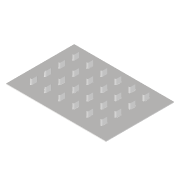
# Autodesk Inventor part: 00_Omniscope_PCB_USBC
Saved by Autodesk Inventor 2022 (Build 260153000, 153)
## iProperties
Created: 2023-05-17
Part Number: 00_Omniscope_PCB_USBC
Material: Generisch
Document SubType Name: Modeling
Designer: diederichbenedict
Density: 1 g/cm^3
Appearance: Vorgabe
Author: diederichbenedict
Autodesk Inventor part; units mm, degrees
(part 1 of 5)
ref_plane "YZ Plane" through (0, 0, 0) normal (1, 0, 0) x (0, 1, 0)
ref_plane "XZ Plane" through (0, 0, 0) normal (0, 1, 0) x (-1, 0, 0)
ref_plane "XY Plane" through (0, 0, 0) normal (0, 0, 1) x (1, 0, 0)
sketch "Skizze5" plane through (0, 0, 0) normal (0, 1, 0) x (-1, 0, 0)
  line L0 (78.8326, 37.2618) -> (79.6226, 37.2618)
  line L1 (79.6226, 37.2618) -> (79.6226, 36.8618)
  line L2 (79.6226, 36.8618) -> (78.8326, 36.8618)
  line L3 (78.8326, 36.8618) -> (78.8326, 37.2618)
  line L4 (76.2926, 37.2618) -> (77.0826, 37.2618)
  line L5 (77.0826, 37.2618) -> (77.0826, 36.8618)
  line L6 (77.0826, 36.8618) -> (76.2926, 36.8618)
  line L7 (76.2926, 36.8618) -> (76.2926, 37.2618)
  line L8 (78.8326, 36.4618) -> (79.6226, 36.4618)
  line L9 (79.6226, 36.4618) -> (79.6226, 36.0618)
  line L10 (79.6226, 36.0618) -> (78.8326, 36.0618)
  line L11 (78.8326, 36.0618) -> (78.8326, 36.4618)
  line L12 (76.2926, 36.4618) -> (77.0826, 36.4618)
  line L13 (77.0826, 36.4618) -> (77.0826, 36.0618)
  line L14 (77.0826, 36.0618) -> (76.2926, 36.0618)
  line L15 (76.2926, 36.0618) -> (76.2926, 36.4618)
  line L16 (78.8326, 35.6618) -> (79.6226, 35.6618)
  line L17 (79.6226, 35.6618) -> (79.6226, 35.2618)
  line L18 (79.6226, 35.2618) -> (78.8326, 35.2618)
  line L19 (78.8326, 35.2618) -> (78.8326, 35.6618)
  line L20 (76.2926, 35.6618) -> (77.0826, 35.6618)
  line L21 (77.0826, 35.6618) -> (77.0826, 35.2618)
  line L22 (77.0826, 35.2618) -> (76.2926, 35.2618)
  line L23 (76.2926, 35.2618) -> (76.2926, 35.6618)
  line L24 (78.8326, 34.8618) -> (79.6226, 34.8618)
  line L25 (79.6226, 34.8618) -> (79.6226, 34.4618)
  line L26 (79.6226, 34.4618) -> (78.8326, 34.4618)
  line L27 (78.8326, 34.4618) -> (78.8326, 34.8618)
  line L28 (76.2926, 34.8618) -> (77.0826, 34.8618)
  line L29 (77.0826, 34.8618) -> (77.0826, 34.4618)
  line L30 (77.0826, 34.4618) -> (76.2926, 34.4618)
  line L31 (76.2926, 34.4618) -> (76.2926, 34.8618)
  line L32 (78.8326, 34.0618) -> (79.6226, 34.0618)
  line L33 (79.6226, 34.0618) -> (79.6226, 33.6618)
  line L34 (79.6226, 33.6618) -> (78.8326, 33.6618)
  line L35 (78.8326, 33.6618) -> (78.8326, 34.0618)
  line L36 (76.2926, 34.0618) -> (77.0826, 34.0618)
  line L37 (77.0826, 34.0618) -> (77.0826, 33.6618)
  line L38 (77.0826, 33.6618) -> (76.2926, 33.6618)
  line L39 (76.2926, 33.6618) -> (76.2926, 34.0618)
  line L40 (78.8326, 33.2618) -> (79.6226, 33.2618)
  line L41 (79.6226, 33.2618) -> (79.6226, 32.8618)
  line L42 (79.6226, 32.8618) -> (78.8326, 32.8618)
  line L43 (78.8326, 32.8618) -> (78.8326, 33.2618)
  line L44 (76.2926, 33.2618) -> (77.0826, 33.2618)
  line L45 (77.0826, 33.2618) -> (77.0826, 32.8618)
  line L46 (77.0826, 32.8618) -> (76.2926, 32.8618)
  line L47 (76.2926, 32.8618) -> (76.2926, 33.2618)
  line L48 (78.8326, 32.4618) -> (79.6226, 32.4618)
  line L49 (79.6226, 32.4618) -> (79.6226, 32.0618)
  line L50 (79.6226, 32.0618) -> (78.8326, 32.0618)
  line L51 (78.8326, 32.0618) -> (78.8326, 32.4618)
  line L52 (76.2926, 32.4618) -> (77.0826, 32.4618)
  line L53 (77.0826, 32.4618) -> (77.0826, 32.0618)
  line L54 (77.0826, 32.0618) -> (76.2926, 32.0618)
  line L55 (76.2926, 32.0618) -> (76.2926, 32.4618)
  line L56 (78.8326, 31.6618) -> (79.6226, 31.6618)
  line L57 (79.6226, 31.6618) -> (79.6226, 31.2618)
  line L58 (79.6226, 31.2618) -> (78.8326, 31.2618)
  line L59 (78.8326, 31.2618) -> (78.8326, 31.6618)
  line L60 (76.2926, 31.6618) -> (77.0826, 31.6618)
  line L61 (77.0826, 31.6618) -> (77.0826, 31.2618)
  line L62 (77.0826, 31.2618) -> (76.2926, 31.2618)
  line L63 (76.2926, 31.2618) -> (76.2926, 31.6618)
  line L64 (77.1576, 38.5368) -> (78.7576, 38.5368)
  line L65 (78.7576, 38.5368) -> (78.7576, 37.8868)
  line L66 (78.7576, 37.8868) -> (77.1576, 37.8868)
  line L67 (77.1576, 37.8868) -> (77.1576, 38.5368)
  line L68 (77.1576, 30.6368) -> (78.7576, 30.6368)
  line L69 (78.7576, 30.6368) -> (78.7576, 29.9868)
  line L70 (78.7576, 29.9868) -> (77.1576, 29.9868)
  line L71 (77.1576, 29.9868) -> (77.1576, 30.6368)
  line L72 (22.0076, 75.1618) -> (22.7976, 75.1618)
  line L73 (22.7976, 75.1618) -> (22.7976, 74.7618)
  line L74 (22.7976, 74.7618) -> (22.0076, 74.7618)
  line L75 (22.0076, 74.7618) -> (22.0076, 75.1618)
  line L76 (19.4676, 75.1618) -> (20.2576, 75.1618)
  line L77 (20.2576, 75.1618) -> (20.2576, 74.7618)
  line L78 (20.2576, 74.7618) -> (19.4676, 74.7618)
  line L79 (19.4676, 74.7618) -> (19.4676, 75.1618)
  line L80 (22.0076, 74.3618) -> (22.7976, 74.3618)
  line L81 (22.7976, 74.3618) -> (22.7976, 73.9618)
  line L82 (22.7976, 73.9618) -> (22.0076, 73.9618)
  line L83 (22.0076, 73.9618) -> (22.0076, 74.3618)
  line L84 (19.4676, 74.3618) -> (20.2576, 74.3618)
  line L85 (20.2576, 74.3618) -> (20.2576, 73.9618)
  line L86 (20.2576, 73.9618) -> (19.4676, 73.9618)
  line L87 (19.4676, 73.9618) -> (19.4676, 74.3618)
  line L88 (22.0076, 73.5618) -> (22.7976, 73.5618)
  line L89 (22.7976, 73.5618) -> (22.7976, 73.1618)
  line L90 (22.7976, 73.1618) -> (22.0076, 73.1618)
  line L91 (22.0076, 73.1618) -> (22.0076, 73.5618)
  line L92 (19.4676, 73.5618) -> (20.2576, 73.5618)
  line L93 (20.2576, 73.5618) -> (20.2576, 73.1618)
  line L94 (20.2576, 73.1618) -> (19.4676, 73.1618)
  line L95 (19.4676, 73.1618) -> (19.4676, 73.5618)
  line L96 (22.0076, 72.7618) -> (22.7976, 72.7618)
  line L97 (22.7976, 72.7618) -> (22.7976, 72.3618)
  line L98 (22.7976, 72.3618) -> (22.0076, 72.3618)
  line L99 (22.0076, 72.3618) -> (22.0076, 72.7618)
  line L100 (19.4676, 72.7618) -> (20.2576, 72.7618)
  line L101 (20.2576, 72.7618) -> (20.2576, 72.3618)
  line L102 (20.2576, 72.3618) -> (19.4676, 72.3618)
  line L103 (19.4676, 72.3618) -> (19.4676, 72.7618)
  line L104 (22.0076, 71.9618) -> (22.7976, 71.9618)
  line L105 (22.7976, 71.9618) -> (22.7976, 71.5618)
  line L106 (22.7976, 71.5618) -> (22.0076, 71.5618)
  line L107 (22.0076, 71.5618) -> (22.0076, 71.9618)
  line L108 (19.4676, 71.9618) -> (20.2576, 71.9618)
  line L109 (20.2576, 71.9618) -> (20.2576, 71.5618)
  line L110 (20.2576, 71.5618) -> (19.4676, 71.5618)
  line L111 (19.4676, 71.5618) -> (19.4676, 71.9618)
  line L112 (22.0076, 71.1618) -> (22.7976, 71.1618)
  line L113 (22.7976, 71.1618) -> (22.7976, 70.7618)
  line L114 (22.7976, 70.7618) -> (22.0076, 70.7618)
  line L115 (22.0076, 70.7618) -> (22.0076, 71.1618)
  line L116 (19.4676, 71.1618) -> (20.2576, 71.1618)
  line L117 (20.2576, 71.1618) -> (20.2576, 70.7618)
  line L118 (20.2576, 70.7618) -> (19.4676, 70.7618)
  line L119 (19.4676, 70.7618) -> (19.4676, 71.1618)
  line L120 (22.0076, 70.3618) -> (22.7976, 70.3618)
  line L121 (22.7976, 70.3618) -> (22.7976, 69.9618)
  line L122 (22.7976, 69.9618) -> (22.0076, 69.9618)
  line L123 (22.0076, 69.9618) -> (22.0076, 70.3618)
  line L124 (19.4676, 70.3618) -> (20.2576, 70.3618)
  line L125 (20.2576, 70.3618) -> (20.2576, 69.9618)
  line L126 (20.2576, 69.9618) -> (19.4676, 69.9618)
  line L127 (19.4676, 69.9618) -> (19.4676, 70.3618)
  line L128 (22.0076, 69.5618) -> (22.7976, 69.5618)
  line L129 (22.7976, 69.5618) -> (22.7976, 69.1618)
  line L130 (22.7976, 69.1618) -> (22.0076, 69.1618)
  line L131 (22.0076, 69.1618) -> (22.0076, 69.5618)
  line L132 (19.4676, 69.5618) -> (20.2576, 69.5618)
  line L133 (20.2576, 69.5618) -> (20.2576, 69.1618)
  line L134 (20.2576, 69.1618) -> (19.4676, 69.1618)
  line L135 (19.4676, 69.1618) -> (19.4676, 69.5618)
  line L136 (20.3326, 76.4368) -> (21.9326, 76.4368)
  line L137 (21.9326, 76.4368) -> (21.9326, 75.7868)
  line L138 (21.9326, 75.7868) -> (20.3326, 75.7868)
  line L139 (20.3326, 75.7868) -> (20.3326, 76.4368)
  line L140 (20.3326, 68.5368) -> (21.9326, 68.5368)
  line L141 (21.9326, 68.5368) -> (21.9326, 67.8868)
  line L142 (21.9326, 67.8868) -> (20.3326, 67.8868)
  line L143 (20.3326, 67.8868) -> (20.3326, 68.5368)
  line L144 (116.3951, 37.3118) -> (117.1851, 37.3118)
  line L145 (117.1851, 37.3118) -> (117.1851, 36.9118)
  line L146 (117.1851, 36.9118) -> (116.3951, 36.9118)
  line L147 (116.3951, 36.9118) -> (116.3951, 37.3118)
  line L148 (113.8551, 37.3118) -> (114.6451, 37.3118)
  line L149 (114.6451, 37.3118) -> (114.6451, 36.9118)
  line L150 (114.6451, 36.9118) -> (113.8551, 36.9118)
  line L151 (113.8551, 36.9118) -> (113.8551, 37.3118)
  line L152 (116.3951, 36.5118) -> (117.1851, 36.5118)
  line L153 (117.1851, 36.5118) -> (117.1851, 36.1118)
  line L154 (117.1851, 36.1118) -> (116.3951, 36.1118)
  line L155 (116.3951, 36.1118) -> (116.3951, 36.5118)
  line L156 (113.8551, 36.5118) -> (114.6451, 36.5118)
  line L157 (114.6451, 36.5118) -> (114.6451, 36.1118)
  line L158 (114.6451, 36.1118) -> (113.8551, 36.1118)
  line L159 (113.8551, 36.1118) -> (113.8551, 36.5118)
  line L160 (116.3951, 35.7118) -> (117.1851, 35.7118)
  line L161 (117.1851, 35.7118) -> (117.1851, 35.3118)
  line L162 (117.1851, 35.3118) -> (116.3951, 35.3118)
  line L163 (116.3951, 35.3118) -> (116.3951, 35.7118)
  line L164 (113.8551, 35.7118) -> (114.6451, 35.7118)
  line L165 (114.6451, 35.7118) -> (114.6451, 35.3118)
  line L166 (114.6451, 35.3118) -> (113.8551, 35.3118)
  line L167 (113.8551, 35.3118) -> (113.8551, 35.7118)
  line L168 (116.3951, 34.9118) -> (117.1851, 34.9118)
  line L169 (117.1851, 34.9118) -> (117.1851, 34.5118)
  line L170 (117.1851, 34.5118) -> (116.3951, 34.5118)
  line L171 (116.3951, 34.5118) -> (116.3951, 34.9118)
  line L172 (113.8551, 34.9118) -> (114.6451, 34.9118)
  line L173 (114.6451, 34.9118) -> (114.6451, 34.5118)
  line L174 (114.6451, 34.5118) -> (113.8551, 34.5118)
  line L175 (113.8551, 34.5118) -> (113.8551, 34.9118)
  line L176 (116.3951, 34.1118) -> (117.1851, 34.1118)
  line L177 (117.1851, 34.1118) -> (117.1851, 33.7118)
  line L178 (117.1851, 33.7118) -> (116.3951, 33.7118)
  line L179 (116.3951, 33.7118) -> (116.3951, 34.1118)
  line L180 (113.8551, 34.1118) -> (114.6451, 34.1118)
  line L181 (114.6451, 34.1118) -> (114.6451, 33.7118)
  line L182 (114.6451, 33.7118) -> (113.8551, 33.7118)
  line L183 (113.8551, 33.7118) -> (113.8551, 34.1118)
  line L184 (116.3951, 33.3118) -> (117.1851, 33.3118)
  line L185 (117.1851, 33.3118) -> (117.1851, 32.9118)
  line L186 (117.1851, 32.9118) -> (116.3951, 32.9118)
  line L187 (116.3951, 32.9118) -> (116.3951, 33.3118)
  line L188 (113.8551, 33.3118) -> (114.6451, 33.3118)
  line L189 (114.6451, 33.3118) -> (114.6451, 32.9118)
  line L190 (114.6451, 32.9118) -> (113.8551, 32.9118)
  line L191 (113.8551, 32.9118) -> (113.8551, 33.3118)
  line L192 (116.3951, 32.5118) -> (117.1851, 32.5118)
  line L193 (117.1851, 32.5118) -> (117.1851, 32.1118)
  line L194 (117.1851, 32.1118) -> (116.3951, 32.1118)
  line L195 (116.3951, 32.1118) -> (116.3951, 32.5118)
  line L196 (113.8551, 32.5118) -> (114.6451, 32.5118)
  line L197 (114.6451, 32.5118) -> (114.6451, 32.1118)
  line L198 (114.6451, 32.1118) -> (113.8551, 32.1118)
  line L199 (113.8551, 32.1118) -> (113.8551, 32.5118)
  line L200 (116.3951, 31.7118) -> (117.1851, 31.7118)
  line L201 (117.1851, 31.7118) -> (117.1851, 31.3118)
  line L202 (117.1851, 31.3118) -> (116.3951, 31.3118)
  line L203 (116.3951, 31.3118) -> (116.3951, 31.7118)
  line L204 (113.8551, 31.7118) -> (114.6451, 31.7118)
  line L205 (114.6451, 31.7118) -> (114.6451, 31.3118)
  line L206 (114.6451, 31.3118) -> (113.8551, 31.3118)
  line L207 (113.8551, 31.3118) -> (113.8551, 31.7118)
  line L208 (114.7201, 38.5868) -> (116.3201, 38.5868)
  line L209 (116.3201, 38.5868) -> (116.3201, 37.9368)
  line L210 (116.3201, 37.9368) -> (114.7201, 37.9368)
  line L211 (114.7201, 37.9368) -> (114.7201, 38.5868)
  line L212 (114.7201, 30.6868) -> (116.3201, 30.6868)
  line L213 (116.3201, 30.6868) -> (116.3201, 30.0368)
  line L214 (116.3201, 30.0368) -> (114.7201, 30.0368)
  line L215 (114.7201, 30.0368) -> (114.7201, 30.6868)
  line L216 (22.0826, 37.3868) -> (22.8726, 37.3868)
  line L217 (22.8726, 37.3868) -> (22.8726, 36.9868)
  line L218 (22.8726, 36.9868) -> (22.0826, 36.9868)
  line L219 (22.0826, 36.9868) -> (22.0826, 37.3868)
  line L220 (19.5426, 37.3868) -> (20.3326, 37.3868)
  line L221 (20.3326, 37.3868) -> (20.3326, 36.9868)
  line L222 (20.3326, 36.9868) -> (19.5426, 36.9868)
  line L223 (19.5426, 36.9868) -> (19.5426, 37.3868)
  line L224 (22.0826, 36.5868) -> (22.8726, 36.5868)
  line L225 (22.8726, 36.5868) -> (22.8726, 36.1868)
  line L226 (22.8726, 36.1868) -> (22.0826, 36.1868)
  line L227 (22.0826, 36.1868) -> (22.0826, 36.5868)
  line L228 (19.5426, 36.5868) -> (20.3326, 36.5868)
  line L229 (20.3326, 36.5868) -> (20.3326, 36.1868)
  line L230 (20.3326, 36.1868) -> (19.5426, 36.1868)
  line L231 (19.5426, 36.1868) -> (19.5426, 36.5868)
  line L232 (22.0826, 35.7868) -> (22.8726, 35.7868)
  line L233 (22.8726, 35.7868) -> (22.8726, 35.3868)
  line L234 (22.8726, 35.3868) -> (22.0826, 35.3868)
  line L235 (22.0826, 35.3868) -> (22.0826, 35.7868)
  line L236 (19.5426, 35.7868) -> (20.3326, 35.7868)
  line L237 (20.3326, 35.7868) -> (20.3326, 35.3868)
  line L238 (20.3326, 35.3868) -> (19.5426, 35.3868)
  line L239 (19.5426, 35.3868) -> (19.5426, 35.7868)
  line L240 (22.0826, 34.9868) -> (22.8726, 34.9868)
  line L241 (22.8726, 34.9868) -> (22.8726, 34.5868)
  line L242 (22.8726, 34.5868) -> (22.0826, 34.5868)
  line L243 (22.0826, 34.5868) -> (22.0826, 34.9868)
  line L244 (19.5426, 34.9868) -> (20.3326, 34.9868)
  line L245 (20.3326, 34.9868) -> (20.3326, 34.5868)
  line L246 (20.3326, 34.5868) -> (19.5426, 34.5868)
  line L247 (19.5426, 34.5868) -> (19.5426, 34.9868)
  line L248 (22.0826, 34.1868) -> (22.8726, 34.1868)
  line L249 (22.8726, 34.1868) -> (22.8726, 33.7868)
  line L250 (22.8726, 33.7868) -> (22.0826, 33.7868)
  line L251 (22.0826, 33.7868) -> (22.0826, 34.1868)
  line L252 (19.5426, 34.1868) -> (20.3326, 34.1868)
  line L253 (20.3326, 34.1868) -> (20.3326, 33.7868)
  line L254 (20.3326, 33.7868) -> (19.5426, 33.7868)
  line L255 (19.5426, 33.7868) -> (19.5426, 34.1868)
  line L256 (22.0826, 33.3868) -> (22.8726, 33.3868)
  line L257 (22.8726, 33.3868) -> (22.8726, 32.9868)
  line L258 (22.8726, 32.9868) -> (22.0826, 32.9868)
  line L259 (22.0826, 32.9868) -> (22.0826, 33.3868)
  line L260 (19.5426, 33.3868) -> (20.3326, 33.3868)
  line L261 (20.3326, 33.3868) -> (20.3326, 32.9868)
  line L262 (20.3326, 32.9868) -> (19.5426, 32.9868)
  line L263 (19.5426, 32.9868) -> (19.5426, 33.3868)
  line L264 (22.0826, 32.5868) -> (22.8726, 32.5868)
  line L265 (22.8726, 32.5868) -> (22.8726, 32.1868)
  line L266 (22.8726, 32.1868) -> (22.0826, 32.1868)
  line L267 (22.0826, 32.1868) -> (22.0826, 32.5868)
  line L268 (19.5426, 32.5868) -> (20.3326, 32.5868)
  line L269 (20.3326, 32.5868) -> (20.3326, 32.1868)
  line L270 (20.3326, 32.1868) -> (19.5426, 32.1868)
  line L271 (19.5426, 32.1868) -> (19.5426, 32.5868)
  line L272 (22.0826, 31.7868) -> (22.8726, 31.7868)
  line L273 (22.8726, 31.7868) -> (22.8726, 31.3868)
  line L274 (22.8726, 31.3868) -> (22.0826, 31.3868)
  line L275 (22.0826, 31.3868) -> (22.0826, 31.7868)
  line L276 (19.5426, 31.7868) -> (20.3326, 31.7868)
  line L277 (20.3326, 31.7868) -> (20.3326, 31.3868)
  line L278 (20.3326, 31.3868) -> (19.5426, 31.3868)
  line L279 (19.5426, 31.3868) -> (19.5426, 31.7868)
  line L280 (20.4076, 38.6618) -> (22.0076, 38.6618)
  line L281 (22.0076, 38.6618) -> (22.0076, 38.0118)
  line L282 (22.0076, 38.0118) -> (20.4076, 38.0118)
  line L283 (20.4076, 38.0118) -> (20.4076, 38.6618)
  line L284 (20.4076, 30.7618) -> (22.0076, 30.7618)
  line L285 (22.0076, 30.7618) -> (22.0076, 30.1118)
  line L286 (22.0076, 30.1118) -> (20.4076, 30.1118)
  line L287 (20.4076, 30.1118) -> (20.4076, 30.7618)
  line L288 (95.7751, 12.7118) -> (94.9851, 12.7118)
  line L289 (94.9851, 12.7118) -> (94.9851, 13.1118)
  line L290 (94.9851, 13.1118) -> (95.7751, 13.1118)
  line L291 (95.7751, 13.1118) -> (95.7751, 12.7118)
  line L292 (98.3151, 12.7118) -> (97.5251, 12.7118)
  line L293 (97.5251, 12.7118) -> (97.5251, 13.1118)
  line L294 (97.5251, 13.1118) -> (98.3151, 13.1118)
  line L295 (98.3151, 13.1118) -> (98.3151, 12.7118)
  line L296 (95.7751, 13.5118) -> (94.9851, 13.5118)
  line L297 (94.9851, 13.5118) -> (94.9851, 13.9118)
  line L298 (94.9851, 13.9118) -> (95.7751, 13.9118)
  line L299 (95.7751, 13.9118) -> (95.7751, 13.5118)
  line L300 (98.3151, 13.5118) -> (97.5251, 13.5118)
  line L301 (97.5251, 13.5118) -> (97.5251, 13.9118)
  line L302 (97.5251, 13.9118) -> (98.3151, 13.9118)
  line L303 (98.3151, 13.9118) -> (98.3151, 13.5118)
  line L304 (95.7751, 14.3118) -> (94.9851, 14.3118)
  line L305 (94.9851, 14.3118) -> (94.9851, 14.7118)
  line L306 (94.9851, 14.7118) -> (95.7751, 14.7118)
  line L307 (95.7751, 14.7118) -> (95.7751, 14.3118)
  line L308 (98.3151, 14.3118) -> (97.5251, 14.3118)
  line L309 (97.5251, 14.3118) -> (97.5251, 14.7118)
  line L310 (97.5251, 14.7118) -> (98.3151, 14.7118)
  line L311 (98.3151, 14.7118) -> (98.3151, 14.3118)
  line L312 (95.7751, 15.1118) -> (94.9851, 15.1118)
  line L313 (94.9851, 15.1118) -> (94.9851, 15.5118)
  line L314 (94.9851, 15.5118) -> (95.7751, 15.5118)
  line L315 (95.7751, 15.5118) -> (95.7751, 15.1118)
  line L316 (98.3151, 15.1118) -> (97.5251, 15.1118)
  line L317 (97.5251, 15.1118) -> (97.5251, 15.5118)
  line L318 (97.5251, 15.5118) -> (98.3151, 15.5118)
  line L319 (98.3151, 15.5118) -> (98.3151, 15.1118)
  line L320 (95.7751, 15.9118) -> (94.9851, 15.9118)
  line L321 (94.9851, 15.9118) -> (94.9851, 16.3118)
  line L322 (94.9851, 16.3118) -> (95.7751, 16.3118)
  line L323 (95.7751, 16.3118) -> (95.7751, 15.9118)
  line L324 (98.3151, 15.9118) -> (97.5251, 15.9118)
  line L325 (97.5251, 15.9118) -> (97.5251, 16.3118)
  line L326 (97.5251, 16.3118) -> (98.3151, 16.3118)
  line L327 (98.3151, 16.3118) -> (98.3151, 15.9118)
  line L328 (95.7751, 16.7118) -> (94.9851, 16.7118)
  line L329 (94.9851, 16.7118) -> (94.9851, 17.1118)
  line L330 (94.9851, 17.1118) -> (95.7751, 17.1118)
  line L331 (95.7751, 17.1118) -> (95.7751, 16.7118)
  line L332 (98.3151, 16.7118) -> (97.5251, 16.7118)
  line L333 (97.5251, 16.7118) -> (97.5251, 17.1118)
  line L334 (97.5251, 17.1118) -> (98.3151, 17.1118)
  line L335 (98.3151, 17.1118) -> (98.3151, 16.7118)
  line L336 (95.7751, 17.5118) -> (94.9851, 17.5118)
  line L337 (94.9851, 17.5118) -> (94.9851, 17.9118)
  line L338 (94.9851, 17.9118) -> (95.7751, 17.9118)
  line L339 (95.7751, 17.9118) -> (95.7751, 17.5118)
  line L340 (98.3151, 17.5118) -> (97.5251, 17.5118)
  line L341 (97.5251, 17.5118) -> (97.5251, 17.9118)
  line L342 (97.5251, 17.9118) -> (98.3151, 17.9118)
  line L343 (98.3151, 17.9118) -> (98.3151, 17.5118)
  line L344 (95.7751, 18.3118) -> (94.9851, 18.3118)
  line L345 (94.9851, 18.3118) -> (94.9851, 18.7118)
  line L346 (94.9851, 18.7118) -> (95.7751, 18.7118)
  line L347 (95.7751, 18.7118) -> (95.7751, 18.3118)
  line L348 (98.3151, 18.3118) -> (97.5251, 18.3118)
  line L349 (97.5251, 18.3118) -> (97.5251, 18.7118)
  line L350 (97.5251, 18.7118) -> (98.3151, 18.7118)
  line L351 (98.3151, 18.7118) -> (98.3151, 18.3118)
  line L352 (97.4501, 11.4368) -> (95.8501, 11.4368)
  line L353 (95.8501, 11.4368) -> (95.8501, 12.0868)
  line L354 (95.8501, 12.0868) -> (97.4501, 12.0868)
  line L355 (97.4501, 12.0868) -> (97.4501, 11.4368)
  line L356 (97.4501, 19.3368) -> (95.8501, 19.3368)
  line L357 (95.8501, 19.3368) -> (95.8501, 19.9868)
  line L358 (95.8501, 19.9868) -> (97.4501, 19.9868)
  line L359 (97.4501, 19.9868) -> (97.4501, 19.3368)
  line L360 (59.8826, 75.0368) -> (60.6726, 75.0368)
  line L361 (60.6726, 75.0368) -> (60.6726, 74.6368)
  line L362 (60.6726, 74.6368) -> (59.8826, 74.6368)
  line L363 (59.8826, 74.6368) -> (59.8826, 75.0368)
  line L364 (57.3426, 75.0368) -> (58.1326, 75.0368)
  line L365 (58.1326, 75.0368) -> (58.1326, 74.6368)
  line L366 (58.1326, 74.6368) -> (57.3426, 74.6368)
  line L367 (57.3426, 74.6368) -> (57.3426, 75.0368)
  line L368 (59.8826, 74.2368) -> (60.6726, 74.2368)
  line L369 (60.6726, 74.2368) -> (60.6726, 73.8368)
  line L370 (60.6726, 73.8368) -> (59.8826, 73.8368)
  line L371 (59.8826, 73.8368) -> (59.8826, 74.2368)
  line L372 (57.3426, 74.2368) -> (58.1326, 74.2368)
  line L373 (58.1326, 74.2368) -> (58.1326, 73.8368)
  line L374 (58.1326, 73.8368) -> (57.3426, 73.8368)
  line L375 (57.3426, 73.8368) -> (57.3426, 74.2368)
  line L376 (59.8826, 73.4368) -> (60.6726, 73.4368)
  line L377 (60.6726, 73.4368) -> (60.6726, 73.0368)
  line L378 (60.6726, 73.0368) -> (59.8826, 73.0368)
  line L379 (59.8826, 73.0368) -> (59.8826, 73.4368)
  line L380 (57.3426, 73.4368) -> (58.1326, 73.4368)
  line L381 (58.1326, 73.4368) -> (58.1326, 73.0368)
  line L382 (58.1326, 73.0368) -> (57.3426, 73.0368)
  line L383 (57.3426, 73.0368) -> (57.3426, 73.4368)
  line L384 (59.8826, 72.6368) -> (60.6726, 72.6368)
  line L385 (60.6726, 72.6368) -> (60.6726, 72.2368)
  line L386 (60.6726, 72.2368) -> (59.8826, 72.2368)
  line L387 (59.8826, 72.2368) -> (59.8826, 72.6368)
  line L388 (57.3426, 72.6368) -> (58.1326, 72.6368)
  line L389 (58.1326, 72.6368) -> (58.1326, 72.2368)
  line L390 (58.1326, 72.2368) -> (57.3426, 72.2368)
  line L391 (57.3426, 72.2368) -> (57.3426, 72.6368)
  line L392 (59.8826, 71.8368) -> (60.6726, 71.8368)
  line L393 (60.6726, 71.8368) -> (60.6726, 71.4368)
  line L394 (60.6726, 71.4368) -> (59.8826, 71.4368)
  line L395 (59.8826, 71.4368) -> (59.8826, 71.8368)
  line L396 (57.3426, 71.8368) -> (58.1326, 71.8368)
  line L397 (58.1326, 71.8368) -> (58.1326, 71.4368)
  line L398 (58.1326, 71.4368) -> (57.3426, 71.4368)
  line L399 (57.3426, 71.4368) -> (57.3426, 71.8368)
  line L400 (59.8826, 71.0368) -> (60.6726, 71.0368)
  line L401 (60.6726, 71.0368) -> (60.6726, 70.6368)
  line L402 (60.6726, 70.6368) -> (59.8826, 70.6368)
  line L403 (59.8826, 70.6368) -> (59.8826, 71.0368)
  line L404 (57.3426, 71.0368) -> (58.1326, 71.0368)
  line L405 (58.1326, 71.0368) -> (58.1326, 70.6368)
  line L406 (58.1326, 70.6368) -> (57.3426, 70.6368)
  line L407 (57.3426, 70.6368) -> (57.3426, 71.0368)
  line L408 (59.8826, 70.2368) -> (60.6726, 70.2368)
  line L409 (60.6726, 70.2368) -> (60.6726, 69.8368)
  line L410 (60.6726, 69.8368) -> (59.8826, 69.8368)
  line L411 (59.8826, 69.8368) -> (59.8826, 70.2368)
  line L412 (57.3426, 70.2368) -> (58.1326, 70.2368)
  line L413 (58.1326, 70.2368) -> (58.1326, 69.8368)
  line L414 (58.1326, 69.8368) -> (57.3426, 69.8368)
  line L415 (57.3426, 69.8368) -> (57.3426, 70.2368)
  line L416 (59.8826, 69.4368) -> (60.6726, 69.4368)
  line L417 (60.6726, 69.4368) -> (60.6726, 69.0368)
  line L418 (60.6726, 69.0368) -> (59.8826, 69.0368)
  line L419 (59.8826, 69.0368) -> (59.8826, 69.4368)
  line L420 (57.3426, 69.4368) -> (58.1326, 69.4368)
  line L421 (58.1326, 69.4368) -> (58.1326, 69.0368)
  line L422 (58.1326, 69.0368) -> (57.3426, 69.0368)
  line L423 (57.3426, 69.0368) -> (57.3426, 69.4368)
  line L424 (58.2076, 76.3118) -> (59.8076, 76.3118)
  line L425 (59.8076, 76.3118) -> (59.8076, 75.6618)
  line L426 (59.8076, 75.6618) -> (58.2076, 75.6618)
  line L427 (58.2076, 75.6618) -> (58.2076, 76.3118)
  line L428 (58.2076, 68.4118) -> (59.8076, 68.4118)
  line L429 (59.8076, 68.4118) -> (59.8076, 67.7618)
  line L430 (59.8076, 67.7618) -> (58.2076, 67.7618)
  line L431 (58.2076, 67.7618) -> (58.2076, 68.4118)
  line L432 (76.7926, 50.4868) -> (76.0026, 50.4868)
  line L433 (76.0026, 50.4868) -> (76.0026, 50.8868)
  line L434 (76.0026, 50.8868) -> (76.7926, 50.8868)
  line L435 (76.7926, 50.8868) -> (76.7926, 50.4868)
  line L436 (79.3326, 50.4868) -> (78.5426, 50.4868)
  line L437 (78.5426, 50.4868) -> (78.5426, 50.8868)
  line L438 (78.5426, 50.8868) -> (79.3326, 50.8868)
  line L439 (79.3326, 50.8868) -> (79.3326, 50.4868)
  line L440 (76.7926, 51.2868) -> (76.0026, 51.2868)
  line L441 (76.0026, 51.2868) -> (76.0026, 51.6868)
  line L442 (76.0026, 51.6868) -> (76.7926, 51.6868)
  line L443 (76.7926, 51.6868) -> (76.7926, 51.2868)
  line L444 (79.3326, 51.2868) -> (78.5426, 51.2868)
  line L445 (78.5426, 51.2868) -> (78.5426, 51.6868)
  line L446 (78.5426, 51.6868) -> (79.3326, 51.6868)
  line L447 (79.3326, 51.6868) -> (79.3326, 51.2868)
  line L448 (76.7926, 52.0868) -> (76.0026, 52.0868)
  line L449 (76.0026, 52.0868) -> (76.0026, 52.4868)
  line L450 (76.0026, 52.4868) -> (76.7926, 52.4868)
  line L451 (76.7926, 52.4868) -> (76.7926, 52.0868)
  line L452 (79.3326, 52.0868) -> (78.5426, 52.0868)
  line L453 (78.5426, 52.0868) -> (78.5426, 52.4868)
  line L454 (78.5426, 52.4868) -> (79.3326, 52.4868)
  line L455 (79.3326, 52.4868) -> (79.3326, 52.0868)
  line L456 (76.7926, 52.8868) -> (76.0026, 52.8868)
  line L457 (76.0026, 52.8868) -> (76.0026, 53.2868)
  line L458 (76.0026, 53.2868) -> (76.7926, 53.2868)
  line L459 (76.7926, 53.2868) -> (76.7926, 52.8868)
  line L460 (79.3326, 52.8868) -> (78.5426, 52.8868)
  line L461 (78.5426, 52.8868) -> (78.5426, 53.2868)
  line L462 (78.5426, 53.2868) -> (79.3326, 53.2868)
  line L463 (79.3326, 53.2868) -> (79.3326, 52.8868)
  line L464 (76.7926, 53.6868) -> (76.0026, 53.6868)
  line L465 (76.0026, 53.6868) -> (76.0026, 54.0868)
  line L466 (76.0026, 54.0868) -> (76.7926, 54.0868)
  line L467 (76.7926, 54.0868) -> (76.7926, 53.6868)
  line L468 (79.3326, 53.6868) -> (78.5426, 53.6868)
  line L469 (78.5426, 53.6868) -> (78.5426, 54.0868)
  line L470 (78.5426, 54.0868) -> (79.3326, 54.0868)
  line L471 (79.3326, 54.0868) -> (79.3326, 53.6868)
  line L472 (76.7926, 54.4868) -> (76.0026, 54.4868)
  line L473 (76.0026, 54.4868) -> (76.0026, 54.8868)
  line L474 (76.0026, 54.8868) -> (76.7926, 54.8868)
  line L475 (76.7926, 54.8868) -> (76.7926, 54.4868)
  line L476 (79.3326, 54.4868) -> (78.5426, 54.4868)
  line L477 (78.5426, 54.4868) -> (78.5426, 54.8868)
  line L478 (78.5426, 54.8868) -> (79.3326, 54.8868)
  line L479 (79.3326, 54.8868) -> (79.3326, 54.4868)
  line L480 (76.7926, 55.2868) -> (76.0026, 55.2868)
  line L481 (76.0026, 55.2868) -> (76.0026, 55.6868)
  line L482 (76.0026, 55.6868) -> (76.7926, 55.6868)
  line L483 (76.7926, 55.6868) -> (76.7926, 55.2868)
  line L484 (79.3326, 55.2868) -> (78.5426, 55.2868)
  line L485 (78.5426, 55.2868) -> (78.5426, 55.6868)
  line L486 (78.5426, 55.6868) -> (79.3326, 55.6868)
  line L487 (79.3326, 55.6868) -> (79.3326, 55.2868)
  line L488 (76.7926, 56.0868) -> (76.0026, 56.0868)
  line L489 (76.0026, 56.0868) -> (76.0026, 56.4868)
  line L490 (76.0026, 56.4868) -> (76.7926, 56.4868)
  line L491 (76.7926, 56.4868) -> (76.7926, 56.0868)
  line L492 (79.3326, 56.0868) -> (78.5426, 56.0868)
  line L493 (78.5426, 56.0868) -> (78.5426, 56.4868)
  line L494 (78.5426, 56.4868) -> (79.3326, 56.4868)
  line L495 (79.3326, 56.4868) -> (79.3326, 56.0868)
  line L496 (78.4676, 49.2118) -> (76.8676, 49.2118)
  line L497 (76.8676, 49.2118) -> (76.8676, 49.8618)
  line L498 (76.8676, 49.8618) -> (78.4676, 49.8618)
  line L499 (78.4676, 49.8618) -> (78.4676, 49.2118)
  line L500 (78.4676, 57.1118) -> (76.8676, 57.1118)
  line L501 (76.8676, 57.1118) -> (76.8676, 57.7618)
  line L502 (76.8676, 57.7618) -> (78.4676, 57.7618)
  line L503 (78.4676, 57.7618) -> (78.4676, 57.1118)
  line L504 (39.1101, 50.4118) -> (38.3201, 50.4118)
  line L505 (38.3201, 50.4118) -> (38.3201, 50.8118)
  line L506 (38.3201, 50.8118) -> (39.1101, 50.8118)
  line L507 (39.1101, 50.8118) -> (39.1101, 50.4118)
  line L508 (41.6501, 50.4118) -> (40.8601, 50.4118)
  line L509 (40.8601, 50.4118) -> (40.8601, 50.8118)
  line L510 (40.8601, 50.8118) -> (41.6501, 50.8118)
  line L511 (41.6501, 50.8118) -> (41.6501, 50.4118)
  line L512 (39.1101, 51.2118) -> (38.3201, 51.2118)
  line L513 (38.3201, 51.2118) -> (38.3201, 51.6118)
  line L514 (38.3201, 51.6118) -> (39.1101, 51.6118)
  line L515 (39.1101, 51.6118) -> (39.1101, 51.2118)
  line L516 (41.6501, 51.2118) -> (40.8601, 51.2118)
  line L517 (40.8601, 51.2118) -> (40.8601, 51.6118)
  line L518 (40.8601, 51.6118) -> (41.6501, 51.6118)
  line L519 (41.6501, 51.6118) -> (41.6501, 51.2118)
  line L520 (39.1101, 52.0118) -> (38.3201, 52.0118)
  line L521 (38.3201, 52.0118) -> (38.3201, 52.4118)
  line L522 (38.3201, 52.4118) -> (39.1101, 52.4118)
  line L523 (39.1101, 52.4118) -> (39.1101, 52.0118)
  line L524 (41.6501, 52.0118) -> (40.8601, 52.0118)
  line L525 (40.8601, 52.0118) -> (40.8601, 52.4118)
  line L526 (40.8601, 52.4118) -> (41.6501, 52.4118)
  line L527 (41.6501, 52.4118) -> (41.6501, 52.0118)
  line L528 (39.1101, 52.8118) -> (38.3201, 52.8118)
  line L529 (38.3201, 52.8118) -> (38.3201, 53.2118)
  line L530 (38.3201, 53.2118) -> (39.1101, 53.2118)
  line L531 (39.1101, 53.2118) -> (39.1101, 52.8118)
  line L532 (41.6501, 52.8118) -> (40.8601, 52.8118)
  line L533 (40.8601, 52.8118) -> (40.8601, 53.2118)
  line L534 (40.8601, 53.2118) -> (41.6501, 53.2118)
  line L535 (41.6501, 53.2118) -> (41.6501, 52.8118)
  line L536 (39.1101, 53.6118) -> (38.3201, 53.6118)
  line L537 (38.3201, 53.6118) -> (38.3201, 54.0118)
  line L538 (38.3201, 54.0118) -> (39.1101, 54.0118)
  line L539 (39.1101, 54.0118) -> (39.1101, 53.6118)
  line L540 (41.6501, 53.6118) -> (40.8601, 53.6118)
  line L541 (40.8601, 53.6118) -> (40.8601, 54.0118)
  line L542 (40.8601, 54.0118) -> (41.6501, 54.0118)
  line L543 (41.6501, 54.0118) -> (41.6501, 53.6118)
  line L544 (39.1101, 54.4118) -> (38.3201, 54.4118)
  line L545 (38.3201, 54.4118) -> (38.3201, 54.8118)
  line L546 (38.3201, 54.8118) -> (39.1101, 54.8118)
  line L547 (39.1101, 54.8118) -> (39.1101, 54.4118)
  line L548 (41.6501, 54.4118) -> (40.8601, 54.4118)
  line L549 (40.8601, 54.4118) -> (40.8601, 54.8118)
  line L550 (40.8601, 54.8118) -> (41.6501, 54.8118)
  line L551 (41.6501, 54.8118) -> (41.6501, 54.4118)
  line L552 (39.1101, 55.2118) -> (38.3201, 55.2118)
  line L553 (38.3201, 55.2118) -> (38.3201, 55.6118)
  line L554 (38.3201, 55.6118) -> (39.1101, 55.6118)
  line L555 (39.1101, 55.6118) -> (39.1101, 55.2118)
  line L556 (41.6501, 55.2118) -> (40.8601, 55.2118)
  line L557 (40.8601, 55.2118) -> (40.8601, 55.6118)
  line L558 (40.8601, 55.6118) -> (41.6501, 55.6118)
  line L559 (41.6501, 55.6118) -> (41.6501, 55.2118)
  line L560 (39.1101, 56.0118) -> (38.3201, 56.0118)
  line L561 (38.3201, 56.0118) -> (38.3201, 56.4118)
  line L562 (38.3201, 56.4118) -> (39.1101, 56.4118)
  line L563 (39.1101, 56.4118) -> (39.1101, 56.0118)
  line L564 (41.6501, 56.0118) -> (40.8601, 56.0118)
  line L565 (40.8601, 56.0118) -> (40.8601, 56.4118)
  line L566 (40.8601, 56.4118) -> (41.6501, 56.4118)
  line L567 (41.6501, 56.4118) -> (41.6501, 56.0118)
  line L568 (40.7851, 49.1368) -> (39.1851, 49.1368)
  line L569 (39.1851, 49.1368) -> (39.1851, 49.7868)
  line L570 (39.1851, 49.7868) -> (40.7851, 49.7868)
  line L571 (40.7851, 49.7868) -> (40.7851, 49.1368)
  line L572 (40.7851, 57.0368) -> (39.1851, 57.0368)
  line L573 (39.1851, 57.0368) -> (39.1851, 57.6868)
  line L574 (39.1851, 57.6868) -> (40.7851, 57.6868)
  line L575 (40.7851, 57.6868) -> (40.7851, 57.0368)
  line L576 (39.2676, 12.7368) -> (38.4776, 12.7368)
  line L577 (38.4776, 12.7368) -> (38.4776, 13.1368)
  line L578 (38.4776, 13.1368) -> (39.2676, 13.1368)
  line L579 (39.2676, 13.1368) -> (39.2676, 12.7368)
  line L580 (41.8076, 12.7368) -> (41.0176, 12.7368)
  line L581 (41.0176, 12.7368) -> (41.0176, 13.1368)
  line L582 (41.0176, 13.1368) -> (41.8076, 13.1368)
  line L583 (41.8076, 13.1368) -> (41.8076, 12.7368)
  line L584 (39.2676, 13.5368) -> (38.4776, 13.5368)
  line L585 (38.4776, 13.5368) -> (38.4776, 13.9368)
  line L586 (38.4776, 13.9368) -> (39.2676, 13.9368)
  line L587 (39.2676, 13.9368) -> (39.2676, 13.5368)
  line L588 (41.8076, 13.5368) -> (41.0176, 13.5368)
  line L589 (41.0176, 13.5368) -> (41.0176, 13.9368)
  line L590 (41.0176, 13.9368) -> (41.8076, 13.9368)
  line L591 (41.8076, 13.9368) -> (41.8076, 13.5368)
  line L592 (39.2676, 14.3368) -> (38.4776, 14.3368)
  line L593 (38.4776, 14.3368) -> (38.4776, 14.7368)
  line L594 (38.4776, 14.7368) -> (39.2676, 14.7368)
  line L595 (39.2676, 14.7368) -> (39.2676, 14.3368)
  line L596 (41.8076, 14.3368) -> (41.0176, 14.3368)
  line L597 (41.0176, 14.3368) -> (41.0176, 14.7368)
  line L598 (41.0176, 14.7368) -> (41.8076, 14.7368)
  line L599 (41.8076, 14.7368) -> (41.8076, 14.3368)
  line L600 (39.2676, 15.1368) -> (38.4776, 15.1368)
  line L601 (38.4776, 15.1368) -> (38.4776, 15.5368)
  line L602 (38.4776, 15.5368) -> (39.2676, 15.5368)
  line L603 (39.2676, 15.5368) -> (39.2676, 15.1368)
  line L604 (41.8076, 15.1368) -> (41.0176, 15.1368)
  line L605 (41.0176, 15.1368) -> (41.0176, 15.5368)
  line L606 (41.0176, 15.5368) -> (41.8076, 15.5368)
  line L607 (41.8076, 15.5368) -> (41.8076, 15.1368)
  line L608 (39.2676, 15.9368) -> (38.4776, 15.9368)
  line L609 (38.4776, 15.9368) -> (38.4776, 16.3368)
  line L610 (38.4776, 16.3368) -> (39.2676, 16.3368)
  line L611 (39.2676, 16.3368) -> (39.2676, 15.9368)
  line L612 (41.8076, 15.9368) -> (41.0176, 15.9368)
  line L613 (41.0176, 15.9368) -> (41.0176, 16.3368)
  line L614 (41.0176, 16.3368) -> (41.8076, 16.3368)
  line L615 (41.8076, 16.3368) -> (41.8076, 15.9368)
  line L616 (39.2676, 16.7368) -> (38.4776, 16.7368)
  line L617 (38.4776, 16.7368) -> (38.4776, 17.1368)
  line L618 (38.4776, 17.1368) -> (39.2676, 17.1368)
  line L619 (39.2676, 17.1368) -> (39.2676, 16.7368)
  line L620 (41.8076, 16.7368) -> (41.0176, 16.7368)
  line L621 (41.0176, 16.7368) -> (41.0176, 17.1368)
  line L622 (41.0176, 17.1368) -> (41.8076, 17.1368)
  line L623 (41.8076, 17.1368) -> (41.8076, 16.7368)
  line L624 (39.2676, 17.5368) -> (38.4776, 17.5368)
  line L625 (38.4776, 17.5368) -> (38.4776, 17.9368)
  line L626 (38.4776, 17.9368) -> (39.2676, 17.9368)
  line L627 (39.2676, 17.9368) -> (39.2676, 17.5368)
  line L628 (41.8076, 17.5368) -> (41.0176, 17.5368)
  line L629 (41.0176, 17.5368) -> (41.0176, 17.9368)
  line L630 (41.0176, 17.9368) -> (41.8076, 17.9368)
  line L631 (41.8076, 17.9368) -> (41.8076, 17.5368)
  line L632 (39.2676, 18.3368) -> (38.4776, 18.3368)
  line L633 (38.4776, 18.3368) -> (38.4776, 18.7368)
  line L634 (38.4776, 18.7368) -> (39.2676, 18.7368)
  line L635 (39.2676, 18.7368) -> (39.2676, 18.3368)
  line L636 (41.8076, 18.3368) -> (41.0176, 18.3368)
  line L637 (41.0176, 18.3368) -> (41.0176, 18.7368)
  line L638 (41.0176, 18.7368) -> (41.8076, 18.7368)
  line L639 (41.8076, 18.7368) -> (41.8076, 18.3368)
  line L640 (40.9426, 11.4618) -> (39.3426, 11.4618)
  line L641 (39.3426, 11.4618) -> (39.3426, 12.1118)
  line L642 (39.3426, 12.1118) -> (40.9426, 12.1118)
  line L643 (40.9426, 12.1118) -> (40.9426, 11.4618)
  line L644 (40.9426, 19.3618) -> (39.3426, 19.3618)
  line L645 (39.3426, 19.3618) -> (39.3426, 20.0118)
  line L646 (39.3426, 20.0118) -> (40.9426, 20.0118)
  line L647 (40.9426, 20.0118) -> (40.9426, 19.3618)
  line L648 (114.8251, 12.6868) -> (114.0351, 12.6868)
  line L649 (114.0351, 12.6868) -> (114.0351, 13.0868)
  line L650 (114.0351, 13.0868) -> (114.8251, 13.0868)
  line L651 (114.8251, 13.0868) -> (114.8251, 12.6868)
  line L652 (117.3651, 12.6868) -> (116.5751, 12.6868)
  line L653 (116.5751, 12.6868) -> (116.5751, 13.0868)
  line L654 (116.5751, 13.0868) -> (117.3651, 13.0868)
  line L655 (117.3651, 13.0868) -> (117.3651, 12.6868)
  line L656 (114.8251, 13.4868) -> (114.0351, 13.4868)
  line L657 (114.0351, 13.4868) -> (114.0351, 13.8868)
  line L658 (114.0351, 13.8868) -> (114.8251, 13.8868)
  line L659 (114.8251, 13.8868) -> (114.8251, 13.4868)
  line L660 (117.3651, 13.4868) -> (116.5751, 13.4868)
  line L661 (116.5751, 13.4868) -> (116.5751, 13.8868)
  line L662 (116.5751, 13.8868) -> (117.3651, 13.8868)
  line L663 (117.3651, 13.8868) -> (117.3651, 13.4868)
  line L664 (114.8251, 14.2868) -> (114.0351, 14.2868)
  line L665 (114.0351, 14.2868) -> (114.0351, 14.6868)
  line L666 (114.0351, 14.6868) -> (114.8251, 14.6868)
  line L667 (114.8251, 14.6868) -> (114.8251, 14.2868)
  line L668 (117.3651, 14.2868) -> (116.5751, 14.2868)
  line L669 (116.5751, 14.2868) -> (116.5751, 14.6868)
  line L670 (116.5751, 14.6868) -> (117.3651, 14.6868)
  line L671 (117.3651, 14.6868) -> (117.3651, 14.2868)
  line L672 (114.8251, 15.0868) -> (114.0351, 15.0868)
  line L673 (114.0351, 15.0868) -> (114.0351, 15.4868)
  line L674 (114.0351, 15.4868) -> (114.8251, 15.4868)
  line L675 (114.8251, 15.4868) -> (114.8251, 15.0868)
  line L676 (117.3651, 15.0868) -> (116.5751, 15.0868)
  line L677 (116.5751, 15.0868) -> (116.5751, 15.4868)
  line L678 (116.5751, 15.4868) -> (117.3651, 15.4868)
  line L679 (117.3651, 15.4868) -> (117.3651, 15.0868)
  line L680 (114.8251, 15.8868) -> (114.0351, 15.8868)
  line L681 (114.0351, 15.8868) -> (114.0351, 16.2868)
  line L682 (114.0351, 16.2868) -> (114.8251, 16.2868)
  line L683 (114.8251, 16.2868) -> (114.8251, 15.8868)
  line L684 (117.3651, 15.8868) -> (116.5751, 15.8868)
  line L685 (116.5751, 15.8868) -> (116.5751, 16.2868)
  line L686 (116.5751, 16.2868) -> (117.3651, 16.2868)
  line L687 (117.3651, 16.2868) -> (117.3651, 15.8868)
  line L688 (114.8251, 16.6868) -> (114.0351, 16.6868)
  line L689 (114.0351, 16.6868) -> (114.0351, 17.0868)
  line L690 (114.0351, 17.0868) -> (114.8251, 17.0868)
  line L691 (114.8251, 17.0868) -> (114.8251, 16.6868)
  line L692 (117.3651, 16.6868) -> (116.5751, 16.6868)
  line L693 (116.5751, 16.6868) -> (116.5751, 17.0868)
  line L694 (116.5751, 17.0868) -> (117.3651, 17.0868)
  line L695 (117.3651, 17.0868) -> (117.3651, 16.6868)
  line L696 (114.8251, 17.4868) -> (114.0351, 17.4868)
  line L697 (114.0351, 17.4868) -> (114.0351, 17.8868)
  line L698 (114.0351, 17.8868) -> (114.8251, 17.8868)
  line L699 (114.8251, 17.8868) -> (114.8251, 17.4868)
  line L700 (117.3651, 17.4868) -> (116.5751, 17.4868)
  line L701 (116.5751, 17.4868) -> (116.5751, 17.8868)
  line L702 (116.5751, 17.8868) -> (117.3651, 17.8868)
  line L703 (117.3651, 17.8868) -> (117.3651, 17.4868)
  line L704 (114.8251, 18.2868) -> (114.0351, 18.2868)
  line L705 (114.0351, 18.2868) -> (114.0351, 18.6868)
  line L706 (114.0351, 18.6868) -> (114.8251, 18.6868)
  line L707 (114.8251, 18.6868) -> (114.8251, 18.2868)
  line L708 (117.3651, 18.2868) -> (116.5751, 18.2868)
  line L709 (116.5751, 18.2868) -> (116.5751, 18.6868)
  line L710 (116.5751, 18.6868) -> (117.3651, 18.6868)
  line L711 (117.3651, 18.6868) -> (117.3651, 18.2868)
  line L712 (116.5001, 11.4118) -> (114.9001, 11.4118)
  line L713 (114.9001, 11.4118) -> (114.9001, 12.0618)
  line L714 (114.9001, 12.0618) -> (116.5001, 12.0618)
  line L715 (116.5001, 12.0618) -> (116.5001, 11.4118)
  line L716 (116.5001, 19.3118) -> (114.9001, 19.3118)
  line L717 (114.9001, 19.3118) -> (114.9001, 19.9618)
  line L718 (114.9001, 19.9618) -> (116.5001, 19.9618)
  line L719 (116.5001, 19.9618) -> (116.5001, 19.3118)
  line L720 (58.0751, 12.8118) -> (57.2851, 12.8118)
  line L721 (57.2851, 12.8118) -> (57.2851, 13.2118)
  line L722 (57.2851, 13.2118) -> (58.0751, 13.2118)
  line L723 (58.0751, 13.2118) -> (58.0751, 12.8118)
  line L724 (60.6151, 12.8118) -> (59.8251, 12.8118)
  line L725 (59.8251, 12.8118) -> (59.8251, 13.2118)
  line L726 (59.8251, 13.2118) -> (60.6151, 13.2118)
  line L727 (60.6151, 13.2118) -> (60.6151, 12.8118)
  line L728 (58.0751, 13.6118) -> (57.2851, 13.6118)
  line L729 (57.2851, 13.6118) -> (57.2851, 14.0118)
  line L730 (57.2851, 14.0118) -> (58.0751, 14.0118)
  line L731 (58.0751, 14.0118) -> (58.0751, 13.6118)
  line L732 (60.6151, 13.6118) -> (59.8251, 13.6118)
  line L733 (59.8251, 13.6118) -> (59.8251, 14.0118)
  line L734 (59.8251, 14.0118) -> (60.6151, 14.0118)
  line L735 (60.6151, 14.0118) -> (60.6151, 13.6118)
  line L736 (58.0751, 14.4118) -> (57.2851, 14.4118)
  line L737 (57.2851, 14.4118) -> (57.2851, 14.8118)
  line L738 (57.2851, 14.8118) -> (58.0751, 14.8118)
  line L739 (58.0751, 14.8118) -> (58.0751, 14.4118)
  line L740 (60.6151, 14.4118) -> (59.8251, 14.4118)
  line L741 (59.8251, 14.4118) -> (59.8251, 14.8118)
  line L742 (59.8251, 14.8118) -> (60.6151, 14.8118)
  line L743 (60.6151, 14.8118) -> (60.6151, 14.4118)
  line L744 (58.0751, 15.2118) -> (57.2851, 15.2118)
  line L745 (57.2851, 15.2118) -> (57.2851, 15.6118)
  line L746 (57.2851, 15.6118) -> (58.0751, 15.6118)
  line L747 (58.0751, 15.6118) -> (58.0751, 15.2118)
  line L748 (60.6151, 15.2118) -> (59.8251, 15.2118)
  line L749 (59.8251, 15.2118) -> (59.8251, 15.6118)
  line L750 (59.8251, 15.6118) -> (60.6151, 15.6118)
  line L751 (60.6151, 15.6118) -> (60.6151, 15.2118)
  line L752 (58.0751, 16.0118) -> (57.2851, 16.0118)
  line L753 (57.2851, 16.0118) -> (57.2851, 16.4118)
  line L754 (57.2851, 16.4118) -> (58.0751, 16.4118)
  line L755 (58.0751, 16.4118) -> (58.0751, 16.0118)
  line L756 (60.6151, 16.0118) -> (59.8251, 16.0118)
  line L757 (59.8251, 16.0118) -> (59.8251, 16.4118)
  line L758 (59.8251, 16.4118) -> (60.6151, 16.4118)
  line L759 (60.6151, 16.4118) -> (60.6151, 16.0118)
  line L760 (58.0751, 16.8118) -> (57.2851, 16.8118)
  line L761 (57.2851, 16.8118) -> (57.2851, 17.2118)
  line L762 (57.2851, 17.2118) -> (58.0751, 17.2118)
  line L763 (58.0751, 17.2118) -> (58.0751, 16.8118)
  line L764 (60.6151, 16.8118) -> (59.8251, 16.8118)
  line L765 (59.8251, 16.8118) -> (59.8251, 17.2118)
  line L766 (59.8251, 17.2118) -> (60.6151, 17.2118)
  line L767 (60.6151, 17.2118) -> (60.6151, 16.8118)
  line L768 (58.0751, 17.6118) -> (57.2851, 17.6118)
  line L769 (57.2851, 17.6118) -> (57.2851, 18.0118)
  line L770 (57.2851, 18.0118) -> (58.0751, 18.0118)
  line L771 (58.0751, 18.0118) -> (58.0751, 17.6118)
  line L772 (60.6151, 17.6118) -> (59.8251, 17.6118)
  line L773 (59.8251, 17.6118) -> (59.8251, 18.0118)
  line L774 (59.8251, 18.0118) -> (60.6151, 18.0118)
  line L775 (60.6151, 18.0118) -> (60.6151, 17.6118)
  line L776 (58.0751, 18.4118) -> (57.2851, 18.4118)
  line L777 (57.2851, 18.4118) -> (57.2851, 18.8118)
  line L778 (57.2851, 18.8118) -> (58.0751, 18.8118)
  line L779 (58.0751, 18.8118) -> (58.0751, 18.4118)
  line L780 (60.6151, 18.4118) -> (59.8251, 18.4118)
  line L781 (59.8251, 18.4118) -> (59.8251, 18.8118)
  line L782 (59.8251, 18.8118) -> (60.6151, 18.8118)
  line L783 (60.6151, 18.8118) -> (60.6151, 18.4118)
  line L784 (59.7501, 11.5368) -> (58.1501, 11.5368)
  line L785 (58.1501, 11.5368) -> (58.1501, 12.1868)
  line L786 (58.1501, 12.1868) -> (59.7501, 12.1868)
  line L787 (59.7501, 12.1868) -> (59.7501, 11.5368)
  line L788 (59.7501, 19.4368) -> (58.1501, 19.4368)
  line L789 (58.1501, 19.4368) -> (58.1501, 20.0868)
  line L790 (58.1501, 20.0868) -> (59.7501, 20.0868)
  line L791 (59.7501, 20.0868) -> (59.7501, 19.4368)
  line L792 (95.6176, 50.3868) -> (94.8276, 50.3868)
  line L793 (94.8276, 50.3868) -> (94.8276, 50.7868)
  line L794 (94.8276, 50.7868) -> (95.6176, 50.7868)
  line L795 (95.6176, 50.7868) -> (95.6176, 50.3868)
  line L796 (98.1576, 50.3868) -> (97.3676, 50.3868)
  line L797 (97.3676, 50.3868) -> (97.3676, 50.7868)
  line L798 (97.3676, 50.7868) -> (98.1576, 50.7868)
  line L799 (98.1576, 50.7868) -> (98.1576, 50.3868)
  line L800 (95.6176, 51.1868) -> (94.8276, 51.1868)
  line L801 (94.8276, 51.1868) -> (94.8276, 51.5868)
  line L802 (94.8276, 51.5868) -> (95.6176, 51.5868)
  line L803 (95.6176, 51.5868) -> (95.6176, 51.1868)
  line L804 (98.1576, 51.1868) -> (97.3676, 51.1868)
  line L805 (97.3676, 51.1868) -> (97.3676, 51.5868)
  line L806 (97.3676, 51.5868) -> (98.1576, 51.5868)
  line L807 (98.1576, 51.5868) -> (98.1576, 51.1868)
  line L808 (95.6176, 51.9868) -> (94.8276, 51.9868)
  line L809 (94.8276, 51.9868) -> (94.8276, 52.3868)
  line L810 (94.8276, 52.3868) -> (95.6176, 52.3868)
  line L811 (95.6176, 52.3868) -> (95.6176, 51.9868)
  line L812 (98.1576, 51.9868) -> (97.3676, 51.9868)
  line L813 (97.3676, 51.9868) -> (97.3676, 52.3868)
  line L814 (97.3676, 52.3868) -> (98.1576, 52.3868)
  line L815 (98.1576, 52.3868) -> (98.1576, 51.9868)
  line L816 (95.6176, 52.7868) -> (94.8276, 52.7868)
  line L817 (94.8276, 52.7868) -> (94.8276, 53.1868)
  line L818 (94.8276, 53.1868) -> (95.6176, 53.1868)
  line L819 (95.6176, 53.1868) -> (95.6176, 52.7868)
  line L820 (98.1576, 52.7868) -> (97.3676, 52.7868)
  line L821 (97.3676, 52.7868) -> (97.3676, 53.1868)
  line L822 (97.3676, 53.1868) -> (98.1576, 53.1868)
  line L823 (98.1576, 53.1868) -> (98.1576, 52.7868)
  line L824 (95.6176, 53.5868) -> (94.8276, 53.5868)
  line L825 (94.8276, 53.5868) -> (94.8276, 53.9868)
  line L826 (94.8276, 53.9868) -> (95.6176, 53.9868)
  line L827 (95.6176, 53.9868) -> (95.6176, 53.5868)
  line L828 (98.1576, 53.5868) -> (97.3676, 53.5868)
  line L829 (97.3676, 53.5868) -> (97.3676, 53.9868)
  line L830 (97.3676, 53.9868) -> (98.1576, 53.9868)
  line L831 (98.1576, 53.9868) -> (98.1576, 53.5868)
  line L832 (95.6176, 54.3868) -> (94.8276, 54.3868)
  line L833 (94.8276, 54.3868) -> (94.8276, 54.7868)
  line L834 (94.8276, 54.7868) -> (95.6176, 54.7868)
  line L835 (95.6176, 54.7868) -> (95.6176, 54.3868)
  line L836 (98.1576, 54.3868) -> (97.3676, 54.3868)
  line L837 (97.3676, 54.3868) -> (97.3676, 54.7868)
  line L838 (97.3676, 54.7868) -> (98.1576, 54.7868)
  line L839 (98.1576, 54.7868) -> (98.1576, 54.3868)
  line L840 (95.6176, 55.1868) -> (94.8276, 55.1868)
  line L841 (94.8276, 55.1868) -> (94.8276, 55.5868)
  line L842 (94.8276, 55.5868) -> (95.6176, 55.5868)
  line L843 (95.6176, 55.5868) -> (95.6176, 55.1868)
  line L844 (98.1576, 55.1868) -> (97.3676, 55.1868)
  line L845 (97.3676, 55.1868) -> (97.3676, 55.5868)
  line L846 (97.3676, 55.5868) -> (98.1576, 55.5868)
  line L847 (98.1576, 55.5868) -> (98.1576, 55.1868)
  line L848 (95.6176, 55.9868) -> (94.8276, 55.9868)
  line L849 (94.8276, 55.9868) -> (94.8276, 56.3868)
  line L850 (94.8276, 56.3868) -> (95.6176, 56.3868)
  line L851 (95.6176, 56.3868) -> (95.6176, 55.9868)
  line L852 (98.1576, 55.9868) -> (97.3676, 55.9868)
  line L853 (97.3676, 55.9868) -> (97.3676, 56.3868)
  line L854 (97.3676, 56.3868) -> (98.1576, 56.3868)
  line L855 (98.1576, 56.3868) -> (98.1576, 55.9868)
  line L856 (97.2926, 49.1118) -> (95.6926, 49.1118)
  line L857 (95.6926, 49.1118) -> (95.6926, 49.7618)
  line L858 (95.6926, 49.7618) -> (97.2926, 49.7618)
  line L859 (97.2926, 49.7618) -> (97.2926, 49.1118)
  line L860 (97.2926, 57.0118) -> (95.6926, 57.0118)
  line L861 (95.6926, 57.0118) -> (95.6926, 57.6618)
  line L862 (95.6926, 57.6618) -> (97.2926, 57.6618)
  line L863 (97.2926, 57.6618) -> (97.2926, 57.0118)
  line L864 (76.9501, 12.8118) -> (76.1601, 12.8118)
  line L865 (76.1601, 12.8118) -> (76.1601, 13.2118)
  line L866 (76.1601, 13.2118) -> (76.9501, 13.2118)
  line L867 (76.9501, 13.2118) -> (76.9501, 12.8118)
  line L868 (79.4901, 12.8118) -> (78.7001, 12.8118)
  line L869 (78.7001, 12.8118) -> (78.7001, 13.2118)
  line L870 (78.7001, 13.2118) -> (79.4901, 13.2118)
  line L871 (79.4901, 13.2118) -> (79.4901, 12.8118)
  line L872 (76.9501, 13.6118) -> (76.1601, 13.6118)
  line L873 (76.1601, 13.6118) -> (76.1601, 14.0118)
  line L874 (76.1601, 14.0118) -> (76.9501, 14.0118)
  line L875 (76.9501, 14.0118) -> (76.9501, 13.6118)
  line L876 (79.4901, 13.6118) -> (78.7001, 13.6118)
  line L877 (78.7001, 13.6118) -> (78.7001, 14.0118)
  line L878 (78.7001, 14.0118) -> (79.4901, 14.0118)
  line L879 (79.4901, 14.0118) -> (79.4901, 13.6118)
  line L880 (76.9501, 14.4118) -> (76.1601, 14.4118)
  line L881 (76.1601, 14.4118) -> (76.1601, 14.8118)
  line L882 (76.1601, 14.8118) -> (76.9501, 14.8118)
  line L883 (76.9501, 14.8118) -> (76.9501, 14.4118)
  line L884 (79.4901, 14.4118) -> (78.7001, 14.4118)
  line L885 (78.7001, 14.4118) -> (78.7001, 14.8118)
  line L886 (78.7001, 14.8118) -> (79.4901, 14.8118)
  line L887 (79.4901, 14.8118) -> (79.4901, 14.4118)
  line L888 (76.9501, 15.2118) -> (76.1601, 15.2118)
  line L889 (76.1601, 15.2118) -> (76.1601, 15.6118)
  line L890 (76.1601, 15.6118) -> (76.9501, 15.6118)
  line L891 (76.9501, 15.6118) -> (76.9501, 15.2118)
  line L892 (79.4901, 15.2118) -> (78.7001, 15.2118)
  line L893 (78.7001, 15.2118) -> (78.7001, 15.6118)
  line L894 (78.7001, 15.6118) -> (79.4901, 15.6118)
  line L895 (79.4901, 15.6118) -> (79.4901, 15.2118)
  line L896 (76.9501, 16.0118) -> (76.1601, 16.0118)
  line L897 (76.1601, 16.0118) -> (76.1601, 16.4118)
  line L898 (76.1601, 16.4118) -> (76.9501, 16.4118)
  line L899 (76.9501, 16.4118) -> (76.9501, 16.0118)
  line L900 (79.4901, 16.0118) -> (78.7001, 16.0118)
  line L901 (78.7001, 16.0118) -> (78.7001, 16.4118)
  line L902 (78.7001, 16.4118) -> (79.4901, 16.4118)
  line L903 (79.4901, 16.4118) -> (79.4901, 16.0118)
  line L904 (76.9501, 16.8118) -> (76.1601, 16.8118)
  line L905 (76.1601, 16.8118) -> (76.1601, 17.2118)
  line L906 (76.1601, 17.2118) -> (76.9501, 17.2118)
  line L907 (76.9501, 17.2118) -> (76.9501, 16.8118)
  line L908 (79.4901, 16.8118) -> (78.7001, 16.8118)
  line L909 (78.7001, 16.8118) -> (78.7001, 17.2118)
  line L910 (78.7001, 17.2118) -> (79.4901, 17.2118)
  line L911 (79.4901, 17.2118) -> (79.4901, 16.8118)
  line L912 (76.9501, 17.6118) -> (76.1601, 17.6118)
  line L913 (76.1601, 17.6118) -> (76.1601, 18.0118)
  line L914 (76.1601, 18.0118) -> (76.9501, 18.0118)
  line L915 (76.9501, 18.0118) -> (76.9501, 17.6118)
  line L916 (79.4901, 17.6118) -> (78.7001, 17.6118)
  line L917 (78.7001, 17.6118) -> (78.7001, 18.0118)
  line L918 (78.7001, 18.0118) -> (79.4901, 18.0118)
  line L919 (79.4901, 18.0118) -> (79.4901, 17.6118)
  line L920 (76.9501, 18.4118) -> (76.1601, 18.4118)
  line L921 (76.1601, 18.4118) -> (76.1601, 18.8118)
  line L922 (76.1601, 18.8118) -> (76.9501, 18.8118)
  line L923 (76.9501, 18.8118) -> (76.9501, 18.4118)
  line L924 (79.4901, 18.4118) -> (78.7001, 18.4118)
  line L925 (78.7001, 18.4118) -> (78.7001, 18.8118)